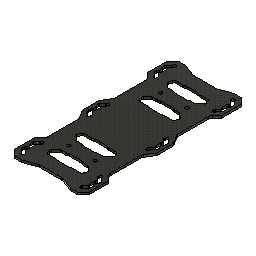
20021-017_payload-deck (Autodesk Fusion 360 design; units mm, degrees)
Autodesk Fusion 360 part; units mm, degrees
note: some values were not read from the file. Set by a fixed rule: the direction of a hole.
sketch "Sketch1" plane through (0, 0, 0) normal (0, 0, 1) x (1, 0, 0)
  line L0 (0, 0) -> (-32.5, 0)
  line L1 (-32.5, 0) -> (-32.5, 7.25)
  line L2 (-32.5, 7.25) -> (-27.5, 15.25)
  line L3 (-27.5, 15.25) -> (-27.5, 44.25)
  line L4 (-27.5, 44.25) -> (-32.5, 49.25)
  line L5 (-32.5, 49.25) -> (-32.5, 66.5)
  line L6 (-32.5, 66.5) -> (-27.5, 71.5)
  line L7 (-27.5, 71.5) -> (-21.2, 71.5)
  line L8 (-21.2, 71.5) -> (-10.3, 67.5)
  line L9 (-10.3, 67.5) -> (0, 67.5)
  line L10 (0, 67.5) -> (0, 0)
  line L11 (-25.8, 50.55) -> (-28.8, 53.55)
  line L12 (-28.8, 53.55) -> (-28.8, 55.125)
  line L13 (-28.8, 55.125) -> (-27.8, 56.125)
  line L14 (-27.8, 56.125) -> (-27.8, 59.625)
  line L15 (-27.8, 59.625) -> (-28.8, 60.625)
  line L16 (-28.8, 60.625) -> (-28.8, 62.2)
  line L17 (-28.8, 62.2) -> (-25.8, 65.2)
  line L18 (-25.8, 65.2) -> (-25.8, 66.2)
  line L19 (-25.8, 50.55) -> (-25.8, 49.55)
  line L20 (-24.5, 49.55) -> (-24.5, 50.55)
  arc A0 (-24.5, 50.55) -> (-27.1, 50.55) centre (-25.8, 50.55) ccw
  line L21 (-27.1, 50.55) -> (-27.1, 49.55)
  arc A1 (-27.1, 49.55) -> (-24.5, 49.55) centre (-25.8, 49.55) ccw
  line L22 (-25.8, 49.55) -> (-25.8, 50.55) construction
  line L23 (-24.8808, 51.4692) -> (-27.8808, 54.4692)
  arc A2 (-27.8808, 54.4692) -> (-29.7192, 52.6308) centre (-28.8, 53.55) ccw
  line L24 (-29.7192, 52.6308) -> (-26.7192, 49.6308)
  arc A3 (-26.7192, 49.6308) -> (-24.8808, 51.4692) centre (-25.8, 50.55) ccw
  line L25 (-25.8, 50.55) -> (-28.8, 53.55) construction
  line L26 (-27.5, 53.55) -> (-27.5, 55.125)
  arc A4 (-27.5, 55.125) -> (-30.1, 55.125) centre (-28.8, 55.125) ccw
  line L27 (-30.1, 55.125) -> (-30.1, 53.55)
  arc A5 (-30.1, 53.55) -> (-27.5, 53.55) centre (-28.8, 53.55) ccw
  line L28 (-28.8, 53.55) -> (-28.8, 55.125) construction
  line L29 (-27.8808, 54.2058) -> (-26.8808, 55.2058)
  arc A6 (-26.8808, 55.2058) -> (-28.7192, 57.0442) centre (-27.8, 56.125) ccw
  line L30 (-28.7192, 57.0442) -> (-29.7192, 56.0442)
  arc A7 (-29.7192, 56.0442) -> (-27.8808, 54.2058) centre (-28.8, 55.125) ccw
  line L31 (-28.8, 55.125) -> (-27.8, 56.125) construction
  line L32 (-26.5, 56.125) -> (-26.5, 59.625)
  arc A8 (-26.5, 59.625) -> (-29.1, 59.625) centre (-27.8, 59.625) ccw
  line L33 (-29.1, 59.625) -> (-29.1, 56.125)
  arc A9 (-29.1, 56.125) -> (-26.5, 56.125) centre (-27.8, 56.125) ccw
  line L34 (-27.8, 56.125) -> (-27.8, 59.625) construction
  line L35 (-26.8808, 60.5442) -> (-27.8808, 61.5442)
  arc A10 (-27.8808, 61.5442) -> (-29.7192, 59.7058) centre (-28.8, 60.625) ccw
  line L36 (-29.7192, 59.7058) -> (-28.7192, 58.7058)
  arc A11 (-28.7192, 58.7058) -> (-26.8808, 60.5442) centre (-27.8, 59.625) ccw
  line L37 (-27.8, 59.625) -> (-28.8, 60.625) construction
  line L38 (-27.5, 60.625) -> (-27.5, 62.2)
  arc A12 (-27.5, 62.2) -> (-30.1, 62.2) centre (-28.8, 62.2) ccw
  line L39 (-30.1, 62.2) -> (-30.1, 60.625)
  arc A13 (-30.1, 60.625) -> (-27.5, 60.625) centre (-28.8, 60.625) ccw
  line L40 (-28.8, 60.625) -> (-28.8, 62.2) construction
  line L41 (-27.8808, 61.2808) -> (-24.8808, 64.2808)
  arc A14 (-24.8808, 64.2808) -> (-26.7192, 66.1192) centre (-25.8, 65.2) ccw
  line L42 (-26.7192, 66.1192) -> (-29.7192, 63.1192)
  arc A15 (-29.7192, 63.1192) -> (-27.8808, 61.2808) centre (-28.8, 62.2) ccw
  line L43 (-28.8, 62.2) -> (-25.8, 65.2) construction
  line L44 (-24.5, 65.2) -> (-24.5, 66.2)
  arc A16 (-24.5, 66.2) -> (-27.1, 66.2) centre (-25.8, 66.2) ccw
  line L45 (-27.1, 66.2) -> (-27.1, 65.2)
  arc A17 (-27.1, 65.2) -> (-24.5, 65.2) centre (-25.8, 65.2) ccw
  line L46 (-25.8, 65.2) -> (-25.8, 66.2) construction
  line L47 (-27.8, 57.875) -> (-27.8, 0) construction
  line L48 (-27.8, 28.9375) -> (0, 28.9375) construction
  line L49 (-28.8, 4.325) -> (-25.8, 7.325) construction
  arc A18 (-27.1, 7.325) -> (-24.5, 7.325) centre (-25.8, 7.325) ccw
  arc A19 (-24.8808, 6.4058) -> (-26.7192, 8.2442) centre (-25.8, 7.325) ccw
  line L50 (-27.8808, 3.4058) -> (-24.8808, 6.4058)
  line L51 (-24.5, 7.325) -> (-24.5, 8.325)
  line L52 (-29.1, 1.75) -> (-29.1, -1.75)
  arc A20 (-24.5, 8.325) -> (-27.1, 8.325) centre (-25.8, 8.325) ccw
  line L53 (-29.7192, 1.8308) -> (-28.7192, 0.8308)
  arc A21 (-30.1, 2.75) -> (-27.5, 2.75) centre (-28.8, 2.75) ccw
  line L54 (-26.8808, 2.6692) -> (-27.8808, 3.6692)
  arc A22 (-27.5, 4.325) -> (-30.1, 4.325) centre (-28.8, 4.325) ccw
  line L55 (-27.8, 1.75) -> (-28.8, 2.75) construction
  arc A23 (-28.7192, 0.8308) -> (-26.8808, 2.6692) centre (-27.8, 1.75) ccw
  arc A24 (-27.8808, 3.6692) -> (-29.7192, 1.8308) centre (-28.8, 2.75) ccw
  line L56 (-26.7192, 8.2442) -> (-29.7192, 5.2442)
  line L57 (-27.1, 8.325) -> (-27.1, 7.325)
  line L58 (-28.8, 2.75) -> (-28.8, 4.325) construction
  line L59 (-27.8, 1.75) -> (-28.8, 2.75)
  line L60 (-28.8, 2.75) -> (-28.8, 4.325)
  arc A25 (-29.7192, 5.2442) -> (-27.8808, 3.4058) centre (-28.8, 4.325) ccw
  line L61 (-27.8, -1.75) -> (-27.8, 1.75) construction
  line L62 (-25.8, 7.325) -> (-25.8, 8.325)
  line L63 (-27.8, -1.75) -> (-27.8, 1.75)
  line L64 (-26.5, -1.75) -> (-26.5, 1.75)
  line L65 (-30.1, 4.325) -> (-30.1, 2.75)
  line L66 (-25.8, 7.325) -> (-25.8, 8.325) construction
  arc A26 (-26.5, 1.75) -> (-29.1, 1.75) centre (-27.8, 1.75) ccw
  line L67 (-27.5, 2.75) -> (-27.5, 4.325)
  line L68 (-28.8, 4.325) -> (-25.8, 7.325)
  arc A27 (-29.1, -1.75) -> (-26.5, -1.75) centre (-27.8, -1.75) ccw
  line L69 (-11.5, 40) -> (0, 40) construction
  line L70 (0, 46.01) -> (-5.375, 46.01)
  line L71 (-5.375, 46.01) -> (-7.1, 46.82)
  line L72 (-7.1, 46.82) -> (-11.94, 46.82)
  line L73 (-11.94, 46.82) -> (-16.71, 51.02)
  line L74 (-16.71, 51.02) -> (-15.215, 55.62)
  line L75 (-15.215, 55.62) -> (-7.165, 55.62)
  line L76 (-7.165, 55.62) -> (-5.35, 56.32)
  line L77 (-5.35, 56.32) -> (0, 56.32)
  line L78 (-16.71, 28.98) -> (-15.215, 24.38)
  line L79 (-7.165, 24.38) -> (-5.35, 23.68)
  line L80 (-11.94, 33.18) -> (-16.71, 28.98)
  line L81 (-5.375, 33.99) -> (-7.1, 33.18)
  line L82 (-7.1, 33.18) -> (-11.94, 33.18)
  line L83 (-5.35, 23.68) -> (0, 23.68)
  line L84 (-15.215, 24.38) -> (-7.165, 24.38)
  line L85 (0, 33.99) -> (-5.375, 33.99)
  point P0 (-32.5, 57.875)
  point P1 (-27.8, 57.875)
  point P2 (-27.8, 0)
  point P3 (-27.8, 0)
  point P4 (-11.5, 40)
  dimension "d1" = 32.5
  dimension "d2" = 27.5
  dimension "d3" = 71.5
  dimension "d4" = 29
  dimension "d5" = 42
  dimension "d6" = 45
  dimension "d7" = 7.25
  dimension "d8" = 10.3
  dimension "d9" = 4
  dimension "d10" = 6.3
  dimension "d11" = 4.7
  dimension "d12" = 3.7
  dimension "d14" = 1
  dimension "d15" = 5.3
  dimension "d16" = 25.8
  dimension "d17" = 5.5
  dimension "d18" = 1.3
  dimension "d21" = 0
  dimension "d22" = -57.875
  dimension "d23" = 11.5
  dimension "d24" = 27.5
  dimension "d25" = 10.31
  dimension "d26" = 8.8
  dimension "d27" = 11.18
  dimension "d28" = 5.35
  dimension "d29" = 7.165
  dimension "d30" = 0.7
  dimension "d31" = 15.215
  dimension "d32" = 16.71
  dimension "d33" = 11.94
  dimension "d34" = 5.375
  dimension "d35" = 7.1
  dimension "d36" = 4.6
  constraint coincident L0.start L10.end
  constraint horizontal L0
  constraint perpendicular L0 L1
  constraint parallel L1 L3
  constraint perpendicular L0 L5
  constraint perpendicular L5 L7
  constraint parallel L0 L9
  constraint perpendicular L0 L10
  constraint coincident L1 L4.end
  constraint equal L4 L6
  constraint coincident L3 L6.end
  constraint perpendicular L6 L11
  constraint perpendicular L11 L13
  constraint parallel L12 L14
  constraint perpendicular L13 L15
  constraint parallel L14 L16
  constraint perpendicular L15 L17
  constraint parallel L16 L18
  constraint equal L11 L17
  constraint equal L12 L16
  constraint equal L13 L15
  constraint midpoint L5 P0
  constraint midpoint L14 P1
  constraint horizontal P0 P1
  constraint vertical L19
  constraint equal L18 L19
  constraint tangent L20 A0
  constraint tangent A0 L21
  constraint parallel L20 L21
  constraint tangent L21 A1
  constraint tangent L20 A1
  constraint coincident L11.start L19.start
  constraint parallel L19 L22
  constraint coincident L19.end A1.centre
  constraint tangent L23 A2
  constraint tangent A2 L24
  constraint parallel L23 L24
  constraint tangent L24 A3
  constraint tangent L23 A3
  constraint coincident L11.end L12.start
  constraint parallel L11 L25
  constraint tangent L26 A4
  constraint tangent A4 L27
  constraint parallel L26 L27
  constraint tangent L27 A5
  constraint tangent L26 A5
  constraint coincident L12.end L13.start
  constraint parallel L12 L28
  constraint tangent L29 A6
  constraint tangent A6 L30
  constraint parallel L29 L30
  constraint tangent L30 A7
  constraint tangent L29 A7
  constraint coincident L13.end L14.start
  constraint parallel L13 L31
  constraint tangent L32 A8
  constraint tangent A8 L33
  constraint parallel L32 L33
  constraint tangent L33 A9
  constraint tangent L32 A9
  constraint coincident L14.end L15.start
  constraint parallel L14 L34
  constraint tangent L35 A10
  constraint tangent A10 L36
  constraint parallel L35 L36
  constraint tangent L36 A11
  constraint tangent L35 A11
  constraint coincident L15.end L16.start
  constraint parallel L15 L37
  constraint tangent L38 A12
  constraint tangent A12 L39
  constraint parallel L38 L39
  constraint tangent L39 A13
  constraint tangent L38 A13
  constraint coincident L16.end L17.start
  constraint parallel L16 L40
  constraint tangent L41 A14
  constraint tangent A14 L42
  constraint parallel L41 L42
  constraint tangent L42 A15
  constraint tangent L41 A15
  constraint coincident L17.end L18.start
  constraint parallel L17 L43
  constraint tangent L44 A16
  constraint tangent A16 L45
  constraint parallel L44 L45
  constraint tangent L45 A17
  constraint tangent L44 A17
  constraint coincident L18.end A16.centre
  constraint parallel L18 L46
  constraint equal A14 A17
  constraint equal A12 A15
  constraint equal A10 A13
  constraint equal A8 A11
  constraint equal A6 A9
  constraint equal A4 A7
  constraint equal A2 A7
  constraint equal A0 A3
  constraint coincident P1 L47.start
  constraint coincident L0 P3
  constraint perpendicular L0 L47
  constraint midpoint L47 L48.start
  constraint coincident L10 L48.end
  constraint perpendicular L10 L48
  constraint coincident P4 L69.start
  constraint coincident L10 L69.end
  constraint perpendicular L10 L69
  constraint coincident L10 L70.start
  constraint perpendicular L10 L70
  constraint perpendicular L10 L72
  constraint perpendicular L10 L75
  constraint coincident L10 L77.end
  constraint perpendicular L10 L77
  constraint symmetric L69 L70.start L85.start
  constraint symmetric L69 L70.end L81.start
  constraint symmetric L69 L71.end L81.end
  constraint symmetric L69 L72.end L80.start
  constraint symmetric L69 L73.end L78.start
  constraint symmetric L69 L74.end L78.end
  constraint symmetric L69 L75.end L79.start
  constraint symmetric L69 L76.end L79.end
  constraint symmetric L69 L77.end L83.end
  measures "d1" distance of L1 L10
  measures "d2" distance of L3 L10
  measures "d3" distance of L0 L7
  measures "d4" distance of L2.end L3.end
  measures "d5" distance of L1.end L4.end
  measures "d6" angle of L6 L7
  measures "d7" distance of L0.end L1.end
  measures "d8" distance of L8.end L9.end
  measures "d9" distance of L7 L9
  measures "d10" distance of L6.end L7.end
  measures "d11" distance of L5 L14
  measures "d12" distance of L5 L16
  measures "d14" distance of L17.end L18.end
  measures "d15" distance of L7 L18.end
  measures "d16" distance of L10 L18
  measures "d17" distance of L12.end L15.end
  measures "d18" radius of A16
  measures "d23" distance of L10 P4
  measures "d24" distance of L9 P4
  measures "d25" distance of L70 L77
  measures "d26" distance of L72 L75
  measures "d27" distance of L9 L77
  measures "d28" distance of L76.end L77.end
  measures "d29" distance of L10 L75.end
  measures "d30" distance of L75 L77
  measures "d31" distance of L10 L74.end
  measures "d32" distance of L10 L73.end
  measures "d33" distance of L10 L72.end
  measures "d34" distance of L70.start L70.end
  measures "d35" distance of L10 L71.end
  measures "d36" distance of L73.end L75
extrude "Extrude1" add sketch "Sketch1" along normal blind 1.95 contours L0 L1 L2 L3 L4 L5 L6 L7 L8 L9 L10 A18 A19 L50 L51 L52 A20 L53 A21 L54 A22 A23 A24 L56 L57 A25 L64 L65 A26 L67 L70 L71 L72 L73 L74 L75 L76 L77 L78 L79 L80 L81 L82 L83 L84 L85 makes body 1
hole "Hole1" at (-11.5, 40, 0) direction (0, 0, 1) diameter 2.9 end through all bodies 1
fillet "Fillet1" radius 1.2 6 edges at (-15.215, 55.62, 0.975) (-16.71, 51.02, 0.975) (-11.94, 46.82, 0.975) (-11.94, 33.18, 0.975) (-16.71, 28.98, 0.975) (-15.215, 24.38, 0.975) on bodies 1
fillet "Fillet2" radius 3 3 edges at (-10.3, 67.5, 0.975) (-27.5, 44.25, 0.975) (-27.5, 15.25, 0.975) on bodies 1
mirror "Mirror1" about plane through (0, 0, 0) normal (0, 1, 0) of bodies 1 makes body 2
mirror "Mirror2" about plane through (0, 0, 0) normal (1, 0, 0) of bodies 1 2 makes body 3 at (9.9548, 10.7329, 0) makes body 4 at (9.9548, -10.7329, 0)
combine "Combine1" operation add target body 1 tool bodies 3 4 2
equation "d1 = ( 65 / 2 ) * 1 mm"
equation "d2 = ( 55 / 2 ) * 1 mm"
equation "d3 = ( 143 / 2 ) * 1 mm"
equation "d7 = ( 14.5 / 2 ) * 1 mm"
equation "d8 = ( 20.6 / 2 ) * 1 mm"
equation "d11 = 3.4 mm + d18"
equation "d12 = 2.4 mm + d18"
equation "d15 = 4 mm + d18"
equation "d16 = ( ( 49 / 2 ) * 1 mm ) + d18"
equation "d23 = ( 23 / 2 ) * 1 mm"
equation "d28 = ( 10.7 / 2 ) * 1 mm"
equation "d29 = ( 14.33 / 2 ) * 1 mm"
equation "d31 = ( 30.43 / 2 ) * 1 mm"
equation "d32 = ( 33.42 / 2 ) * 1 mm"
equation "d33 = ( 23.88 / 2 ) * 1 mm"
equation "d34 = ( 10.75 / 2 ) * 1 mm"
equation "d35 = ( 14.2 / 2 ) * 1 mm"
named bodies: "20021-017_payload-deck"
